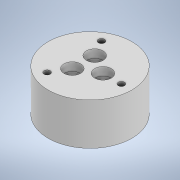
# Autodesk Inventor part: EF1
Saved by Autodesk Inventor 2022 (Build 260153000, 153)
## iProperties
Created: 2022-05-31
Part Number: EF1
Material: Generic
Document SubType Name: Modeling
Designer: Asus
Density: 1 g/cm^3
Appearance: Default
Author: Asus
Autodesk Inventor part; units mm, degrees
sketch "Sketch1" plane through (0, 0, 0) normal (0, 1, 0) x (-1, 0, 0)
  circle A0 centre (0, 0) radius 20
  dimension "d0" = 40
  constraints: 1 centre point, 1 coincident
  measures "d0" diameter of A0
extrude "Extrusion1" add sketch "Sketch1" along normal blind 30
sketch "Sketch2" plane through (0, 30, 0) normal (0, 1, 0) x (1, 0, 0)
  circle A0 centre (0, 0) radius 10
  dimension "d3" = 20
  constraints: 1 centre point, 1 coincident
  measures "d3" diameter of A0
extrude "Extrusion2" add sketch "Sketch2" along normal blind 60
sketch "Sketch3" plane through (0, 90, 0) normal (0, 1, 0) x (1, 0, 0)
  circle A0 centre (0, 0) radius 10 projected
  circle A1 centre (0, 0) radius 10
  circle A2 centre (0, 0) radius 6
  dimension "d6" = 20
  dimension "d7" = 12
  constraints: 2 centre point, 2 coincident
  measures "d6" diameter of A1
  measures "d7" diameter of A2
extrude "Extrusion3" cut sketch "Sketch3" against normal blind 16
sketch "Sketch4" plane through (0, 0, 0) normal (0, -1, 0) x (1, 0, 0)
  circle A0 centre (0, 0) radius 2
  line L0 (1.5, 1.3229) -> (1.5, -1.3229)
  dimension "d10" = 4
  dimension "d11" = 3.5
  constraints: 2 end point, 2 point on circle, 1 centre point, 1 coincident, 1 vertical
  measures "d10" diameter of A0
extrude "Extrusion4" cut sketch "Sketch4" against normal blind 10 contours L0 A0 picked at (-0.0779, 0.6608)
fillet "Fillet1" radius 7 1 edges at (-10, 30, 0)
fillet "Fillet2" radius 7 1 edges at (20, 30, 0)
fillet "Fillet3" radius 4 1 edges at (-6, 90, 0)
ref_plane "Work Plane1" through (6, 0, 0) normal (1, 0, 0) x (0, 1, 0)
ref_plane "Work Plane2" through (-6, 0, 0) normal (1, 0, 0) x (0, 1, 0)
ref_plane "Work Plane3" through (10, 0, 0) normal (1, 0, 0) x (0, 1, 0)
sketch "Sketch7" plane through (10, 0, 0) normal (1, 0, 0) x (0, 1, 0)
  line L0 (57, 6.8) -> (37.3, 6.8)
  line L1 (37.3, 6.8) -> (37.3, -6.8)
  line L2 (37.3, -6.8) -> (57, -6.8)
  line L3 (57, -6.8) -> (57, 6.8)
  line L4 (-9.9161, 0) -> (11.1387, 0)
  line L5 (74, 10) -> (74, -10) projected
  line L6 (37.3, -6.8) -> (32.3, -6.8)
  line L7 (37.3, 4) -> (31.3, 4)
  line L8 (31.3, 4) -> (31.3, -4)
  line L9 (31.3, -4) -> (37.3, -4)
  line L10 (37.3, -4) -> (37.3, 4)
  point P0 (0, 0)
  dimension "d26" = 6.8
  dimension "d27" = 13.6
  dimension "d28" = 19.7
  dimension "d29" = 17
  dimension "d30" = 0
  dimension "d31" = 5
  dimension "d32" = 6
  dimension "d33" = 8
  dimension "d38" = 4
  dimension "d39" = 0
  constraints: 20 end point, 4 horizontal, 4 parallel, 2 perpendicular
  measures "d26" distance between parallel lines of L4 L2
  measures "d27" distance of L2.end L0.start
  measures "d28" distance of L1.end L2.end
  measures "d29" distance between parallel lines of L5 L3
  measures "d30" distance from line of point (0, 0) L4
  measures "d31" distance of L1.end L6.end
  measures "d32" distance of L8.end L9.end
  measures "d33" distance of L7.end L8.end
  measures "d38" distance between parallel lines of L4 L9
  measures "d39" distance between parallel lines of L1 L10
extrude "Extrusion6" cut sketch "Sketch7" along normal blind 2 and the other way blind 4
ref_plane "Work Plane4" through (12, 31.3, 4) normal (0.7071, 0.7071, 0) x (0, 0, -1)
sketch "Sketch8" plane through (12, 31.3, 4) normal (0.7071, 0.7071, 0) x (0, 0, -1)
  line L0 (8, 4.2426) -> (8, 0) projected
  line L1 (8, 4.3868) -> (0, 4.3868)
  line L2 (0, 4.3868) -> (0, -12.1132)
  line L3 (0, -12.1132) -> (8, -12.1132)
  line L4 (8, -12.1132) -> (8, 4.3868)
  ellipse E0 centre (4, 26.6579) end of major axis (14, 26.6579) minor radius 7.0711 (-2.8, 21.4733) -> (10.8, 21.4733) ccw projected
  point P0 (4, -13.6472)
  point P1 (8, 4.2426)
  dimension "d41" = 8
  dimension "d42" = 16.5
  dimension "d52" = 22.2711
  constraints: 8 end point, 2 parallel, 1 horizontal, 1 perpendicular, 1 point on line, 1 other
  measures "d41" distance of L1.start L1.end
  measures "d42" distance of L1.end L2.end
  measures "d52" distance from line of point (4, 26.658) L1
extrude "Extrusion7" cut sketch "Sketch8" along normal blind 3 and the other way blind 4.2
ref_plane "Work Plane5" through (0, 0, 6) normal (0, 0, 1) x (1, 0, 0)
sketch "Sketch9" plane through (0, 0, 6) normal (0, 0, 1) x (1, 0, 0)
  circle A0 centre (0, 79) radius 1.5
  line L0 (-10, 74) -> (10, 74) projected
  point P0 (0, 0)
  dimension "d48" = 3
  dimension "d49" = 5
  constraints: 1 centre point
  measures "d48" diameter of A0
  measures "d49" distance from line of L0 A0.centre
extrude "Extrusion8" cut sketch "Sketch9" against normal blind 3
mirror "Mirror2" about plane through (0, 0, 0) normal (0, 0, 1) of "Extrusion8"
sketch "Sketch10" plane through (0, 0, 0) normal (0, -1, 0) x (1, 0, 0)
  circle A0 centre (0, 0) radius 9.5
  dimension "d53" = 19
  constraints: 1 centre point, 1 coincident
  measures "d53" diameter of A0
extrude "Extrusion9" cut sketch "Sketch10" against normal blind 12
sketch "Sketch11" plane through (0, 0, 0) normal (0, -1, 0) x (1, 0, 0)
  circle A0 centre (0, 0) radius 9.5 projected
  circle A1 centre (0, 0) radius 11.5
  dimension "d56" = 23
  constraints: 1 centre point, 1 coincident
  measures "d56" diameter of A1
extrude "Extrusion10" cut sketch "Sketch11" against normal blind 6.5
ref_plane "Work Plane6" through (-20, 0, 0) normal (1, 0, 0) x (0, 1, 0)
sketch "Sketch12" plane through (-20, 0, 0) normal (1, 0, 0) x (0, 1, 0)
  line L0 (0, -20) -> (0, 20) projected
  line L1 (0, -11.1927) -> (6.5, -11.1927)
  line L2 (6.5, -11.1927) -> (6.5, 10.8073)
  line L3 (6.5, 10.8073) -> (0, 10.8073)
  line L4 (0, 10.8073) -> (0, -11.1927)
  circle A0 centre (3.25, 0) radius 1.95
  circle A1 centre (8.75, 0) radius 1.95
  point P0 (0, 0)
  dimension "d60" = 22
  dimension "d61" = 3.9
  dimension "d62" = 6.5
  dimension "d63" = 3.25
  dimension "d64" = 0
  dimension "d65" = 3.9
  dimension "d66" = 5.5
  constraints: 8 end point, 2 centre point, 2 parallel, 1 horizontal, 1 perpendicular, 1 point on line
  measures "d60" distance of L1.end L2.end
  measures "d61" diameter of A0
  measures "d62" distance of L1.start L1.end
  measures "d63" distance from line of L0 A0.centre
  measures "d64" vertical distance of point (0, 0) A0.centre
  measures "d65" diameter of A1
  measures "d66" distance of A0.centre A1.centre
extrude "Extrusion11" cut sketch "Sketch12" along normal blind 18 contours A0 | A1
sketch "Sketch13" plane through (-20, 0, 0) normal (1, 0, 0) x (0, 1, 0)
  line L0 (0, -4) -> (13, -4)
  line L1 (13, -4) -> (13, 4)
  line L2 (13, 4) -> (0, 4)
  line L3 (0, 4) -> (0, -4)
  point P0 (0, 0)
  dimension "d70" = 8
  dimension "d71" = 4
  dimension "d72" = 13
  constraints: 8 end point, 2 parallel, 1 horizontal, 1 perpendicular
  measures "d70" distance between parallel lines of L2 L0
  measures "d71" distance from line of point (0, 0) L2
  measures "d72" distance of L0.start L0.end
extrude "Extrusion12" cut sketch "Sketch13" along normal blind 2
sketch "Sketch14" plane through (0, 12, 0) normal (0, -1, 0) x (1, 0, 0)
  circle A0 centre (0, 0) radius 6.2
  line L0 (0, 0) -> (7.6867, 0)
  line L1 (0, 0) -> (-3.9527, 6.8463)
  line L2 (0, 0) -> (-3.8209, -6.618)
  circle A1 centre (-3.1, 5.3694) radius 1.45
  circle A2 centre (-3.1, -5.3694) radius 1.45
  circle A3 centre (6.2, 0) radius 1.45
  dimension "d75" = 12.4
  dimension "d76" = 120
  dimension "d77" = 120
  dimension "d79" = 2.9
  dimension "d80" = 2.9
  dimension "d81" = 2.9
  constraints: 6 end point, 4 centre point, 3 point on circle, 3 point on line, 1 coincident, 1 horizontal
  measures "d75" diameter of A0
  measures "d76" angle of L0 L1
  measures "d77" angle of L2 L1
  measures "d79" diameter of A2
  measures "d80" diameter of A1
  measures "d81" diameter of A3
extrude "Extrusion13" cut sketch "Sketch14" against normal blind 12 contours L0 A3 A0 | L0 A3 A0 | A0 A3 L0 | A0 A3 L0 | A1 L1 A0 | A0 L1 A1 | A2 A0 | A0 L2 A2 | L1 A1 A0 | A0 A1 L1 | A0 A2 L2
sketch "Sketch15" plane through (0, 0, 0) normal (1, 0, 0) x (0, 1, 0)
  line L0 (95, -20.5708) -> (0, -20.5708)
  line L1 (0, -20.5708) -> (0, 21.1406)
  line L2 (0, 21.1406) -> (95, 21.1406)
  line L3 (95, 21.1406) -> (95, -20.5708)
  line L4 (20, -20.5708) -> (20, 21.1406)
  point P0 (0, 0)
  dimension "d84" = 20
  dimension "d85" = 41.7114
  dimension "d86" = 95
  constraints: 10 end point, 2 parallel, 2 point on line, 1 horizontal, 1 perpendicular, 1 vertical
  measures "d84" distance between parallel lines of L1 L4
  measures "d85" distance of L0.end L1.end
  measures "d86" distance of L0.start L0.end
extrude "Extrusion14" cut sketch "Sketch15" along normal mid plane 40 contours L0 L4 L2 L3
sketch "Sketch16" plane through (0, 20, 0) normal (0, 1, 0) x (1, 0, 0)
  line L0 (18.2415, 4.1496) -> (17.0061, 4.1496)
  line L1 (17.0061, 4.1496) -> (17.0061, -4.2806)
  line L2 (17.0061, -4.2806) -> (18.2415, -4.2806)
  line L3 (18.2415, -4.2806) -> (18.2415, 4.1496)
  point P0 (0, 0)
  constraints: 8 end point, 2 parallel, 1 horizontal, 1 perpendicular
extrude "Extrusion15" add sketch "Sketch16" against normal blind 3
sketch "Sketch17" plane through (0, 20, 0) normal (0, 1, 0) x (1, 0, 0)
  circle A0 centre (0, 0) radius 15
  circle A1 centre (-3.1, -5.3694) radius 1.45 projected
  circle A2 centre (-3.1, -5.3694) radius 4
  circle A3 centre (-3.1, 5.3694) radius 1.45 projected
  circle A4 centre (-3.1, 5.3694) radius 4
  circle A5 centre (6.2, 0) radius 1.45 projected
  circle A6 centre (6.2, 0) radius 4
  dimension "d91" = 30
  dimension "d92" = 8
  dimension "d93" = 8
  dimension "d94" = 8
  constraints: 4 centre point, 4 coincident
  measures "d91" diameter of A0
  measures "d92" diameter of A6
  measures "d93" diameter of A2
  measures "d94" diameter of A4
extrude "Extrusion16" cut sketch "Sketch17" against normal blind 4 contours A2 | A4 | A6
sketch "Sketch18" plane through (0, 20, 0) normal (0, 1, 0) x (1, 0, 0)
  circle A0 centre (0, 0) radius 15
  line L0 (0, 0) -> (18.2122, 0)
  line L1 (0, 0) -> (-8.7364, -15.1318)
  line L2 (0, 0) -> (-8.9499, 15.5016)
  circle A1 centre (15, 0) radius 1.5
  circle A2 centre (-7.5, -12.9904) radius 1.5
  circle A3 centre (-7.5, 12.9904) radius 1.5
  dimension "d97" = 30
  dimension "d98" = 120
  dimension "d99" = 120
  dimension "d100" = 3
  dimension "d101" = 3
  dimension "d102" = 3
  constraints: 6 end point, 4 centre point, 3 point on circle, 3 point on line, 1 coincident, 1 horizontal
  measures "d97" diameter of A0
  measures "d98" angle of L2 L1
  measures "d99" angle of L0 L2
  measures "d100" diameter of A3
  measures "d101" diameter of A2
  measures "d102" diameter of A1
extrude "Extrusion17" cut sketch "Sketch18" against normal blind 40 contours L0 A1 A0 | L0 A1 A0 | A0 A1 L0 | A0 A1 L0 | A3 L2 A0 | A0 L2 A3 | A2 L1 A0 | A0 L1 A2 | L2 A3 A0 | A0 A3 L2 | L1 A2 A0 | A0 A2 L1
sketch "Sketch19" plane through (0, 0, 0) normal (0, -1, 0) x (1, 0, 0)
  circle A0 centre (-7.5, -12.9904) radius 1.5 projected
  circle A1 centre (-7.5, -12.9904) radius 3.5
  circle A2 centre (15, 0) radius 1.5 projected
  circle A3 centre (15, 0) radius 3.5
  circle A4 centre (-7.5, 12.9904) radius 1.5 projected
  circle A5 centre (-7.5, 12.9904) radius 3.5
  point P0 (0, 0)
  dimension "d105" = 7
  dimension "d106" = 7
  dimension "d107" = 7
  constraints: 3 centre point, 3 coincident
  measures "d105" diameter of A5
  measures "d106" diameter of A1
  measures "d107" diameter of A3
extrude "Extrusion18" cut sketch "Sketch19" against normal blind 5
body "Solid1"
